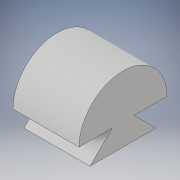
# Autodesk Inventor part: knee ball
Saved by Autodesk Inventor 2019 (Build 230136000, 136)
## iProperties
Created: 2018-07-06
Part Number: knee ball
Material: Generic
Document SubType Name: Modeling
Designer: HIVE
Density: 1 g/cm^3
Appearance: Default
legDiam: 40.000 mm
clearance: 1.000 mm
hingeHoleDiam: 10.000 mm
kneeBallBaseW: 30.000 mm
kneeBallBaseL: 30.000 mm
kneeBallBaseH: 10.000 mm
kneeBallLocationUp: 10.000 mm
kneeBallDepth: 20.000 mm
kneeBallLocationExtend: 20.000 mm
Author: HIVE
Autodesk Inventor part; units mm, degrees
ref_plane "YZ Plane" through (0, 0, 0) normal (1, 0, 0) x (0, 1, 0)
ref_plane "XZ Plane" through (0, 0, 0) normal (0, 1, 0) x (-1, 0, 0)
ref_plane "XY Plane" through (0, 0, 0) normal (0, 0, 1) x (1, 0, 0)
sketch "Sketch1" plane through (0, 0, 0) normal (1, 0, 0) x (0, 1, 0)
  line L0 (0, 15) -> (0, -15)
  line L1 (0, -15) -> (10, -5)
  line L2 (10, -5) -> (10, -20)
  arc A0 (10, -20) -> (10, 20) centre (10, 0) ccw
  line L3 (10, 20) -> (10, 5)
  line L4 (10, 5) -> (0, 15)
  line L5 (0, 0) -> (1.9219, 0) construction
  dimension "d0" = 45
  dimension "d1" = 45
  dimension "kneeBallBaseW" = 30
  dimension "d3" = 20
  dimension "kneeBallBaseH" = 10
  constraints: 12 end point, 4 point on line, 2 midpoint, 2 point on circle, 1 centre point, 1 collinear, 1 horizontal, 1 parallel, 1 vertical
  measures "d0" angle of L3 L4
  measures "d1" angle of L2 L1
  measures "kneeBallBaseW" distance of L0.start L0.end
  measures "d3" radius of A0
  measures "kneeBallBaseH" distance between parallel lines of L0 L2
extrude "Extrusion2" add sketch "Sketch1" along normal blind 30
equation "\"kneeBallBaseW\" = kneeBallBaseL"
equation "\"d3\" = 0.666667 * kneeBallBaseL"
equation "\"d7\" = kneeBallBaseL"
equation "\"legDiam\" = 40"
equation "\"clearance\" = 1"
equation "\"hingeHoleDiam\" = 10"
equation "\"kneeBallLocationUp\" = 10"
equation "\"kneeBallDepth\" = 20"
equation "\"kneeBallLocationExtend\" = 20"
equation "\"kneeBallBaseL\" = 30"
body "Solid2"
